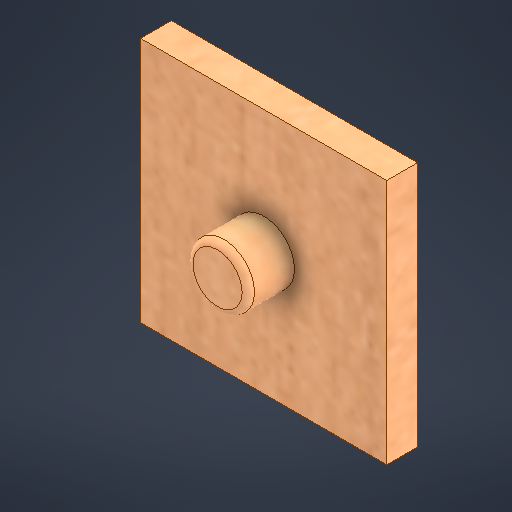
# Autodesk Inventor part: base
Saved by Autodesk Inventor 2026.4 (Build 304435000, 435)
## iProperties
Created: 2026-08-27
Part Number: base
Material: Genérico
Document SubType Name: Modeling
Designer: Matheus
Density: 1 g/cm^3
Appearance: Cerejeira - Natural com pouco brilho
Author: Matheus
Autodesk Inventor part; units mm, degrees
ref_plane "YZ Plane" through (0, 0, 0) normal (1, 0, 0) x (0, 1, 0)
ref_plane "XZ Plane" through (0, 0, 0) normal (0, 1, 0) x (-1, 0, 0)
ref_plane "XY Plane" through (0, 0, 0) normal (0, 0, 1) x (1, 0, 0)
sketch "Esboço1" plane through (0, 0, 0) normal (0, 0, 1) x (1, 0, 0)
  line L0 (0, 0) -> (40, 0)
  line L1 (40, 0) -> (40, 40)
  line L2 (40, 40) -> (0, 40)
  line L3 (0, 40) -> (0, 0)
  dimension "d0" = 40
  dimension "d1" = 40
  constraints: 8 end point, 2 parallel, 1 horizontal, 1 perpendicular
  measures "d0" distance of L1.end L2.end
  measures "d1" distance of L0.end L1.end
extrude "Extrusão1" add sketch "Esboço1" along normal mid plane 5
sketch "Esboço2" plane through (0, 0, 2.5) normal (0, 0, 1) x (1, 0, 0)
  line L0 (0, 40) -> (0, 0) projected
  line L1 (0, 20) -> (40, 20)
  line L2 (40, 0) -> (40, 40) projected
  circle A0 centre (20, 20) radius 5
  dimension "d6" = 10
  constraints: 3 midpoint, 2 end point, 1 centre point
  measures "d6" diameter of A0
extrude "Extrusão2" add sketch "Esboço2" along normal blind 7.5
fillet "Arredondamento1" radius 1 1 edges at (15, 20, 10)
